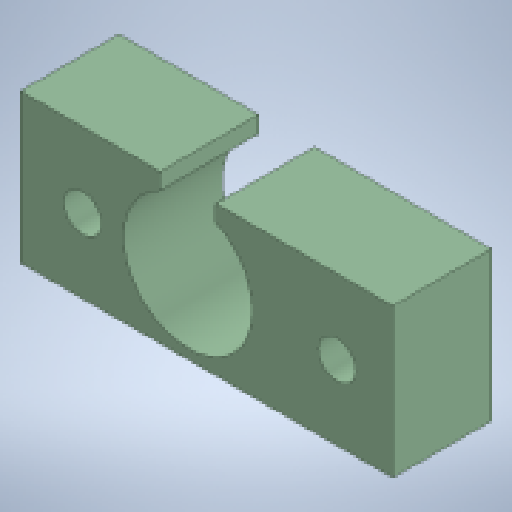
# Autodesk Inventor part: Pod
Saved by Autodesk Inventor 2023.2 (Build 272271000, 271)
## iProperties
Created: 2023-03-29
Part Number: Pod
Material: UHMW, White
Document SubType Name: Modeling
Designer: Nathan Cai
Density: 0.94 g/cm^3
Appearance: Rubber - Green
Author: Nathan Cai
Autodesk Inventor part; units mm, degrees
ref_plane "YZ Plane" through (0, 0, 0) normal (1, 0, 0) x (0, 1, 0)
ref_plane "XZ Plane" through (0, 0, 0) normal (0, 1, 0) x (-1, 0, 0)
ref_plane "XY Plane" through (0, 0, 0) normal (0, 0, 1) x (1, 0, 0)
sketch "Sketch1" plane through (0, 0, 0) normal (0, 0, 1) x (1, 0, 0)
  circle A0 centre (0, 0) radius 11
  line L0 (0, 0) -> (-18, 0) construction
  circle A1 centre (-18, 0) radius 3.175
  circle A2 centre (-18, 0) radius 38.1 construction
  circle A3 centre (25.4, 0) radius 1.7526 construction
  circle A4 centre (25.4, 0) radius 3.175
  line L1 (-23.8125, 12.7) -> (14.2875, 12.7)
  line L2 (14.2875, 12.7) -> (14.2875, -12.7)
  line L3 (14.2875, -12.7) -> (-23.8125, -12.7)
  line L4 (-23.8125, -12.7) -> (-23.8125, 12.7)
  line L5 (-23.8125, 12.7) -> (14.2875, -12.7) construction
  line L6 (14.2875, 12.7) -> (-23.8125, -12.7) construction
  line L7 (-9.525, -9.525) -> (9.525, -9.525) construction
  line L8 (9.525, -9.525) -> (9.525, 9.525) construction
  line L9 (9.525, 9.525) -> (-9.525, 9.525) construction
  line L10 (-9.525, 9.525) -> (-9.525, -9.525) construction
  line L11 (-9.525, -9.525) -> (9.525, 9.525) construction
  line L12 (9.525, -9.525) -> (-9.525, 9.525) construction
  circle A5 centre (-9.525, 9.525) radius 1.7526
  circle A6 centre (9.525, 9.525) radius 1.7526
  circle A7 centre (-9.525, -9.525) radius 1.7526
  circle A8 centre (9.525, -9.525) radius 1.7526
  point P0 (-4.7625, 0)
  dimension "d0" = 22
  dimension "d1" = 18
  dimension "d2" = 6.35
  dimension "d3" = 76.2
  dimension "d4" = 3.5052
  dimension "d5" = 25.4
  dimension "d6" = 6.35
  dimension "d7" = 38.1
  dimension "d8" = 25.4
  dimension "d16" = 4.7625
  dimension "d18" = 19.05
  dimension "d19" = 19.05
  dimension "d20" = 3.5052
  dimension "d23" = 19.05
  dimension "d26" = 19.05
  constraints: 26 end point, 9 centre point, 5 coincident, 4 horizontal, 4 midpoint, 4 parallel, 2 perpendicular, 2 point on line, 1 vertical, 6 other
  measures "d0" diameter of A0
  measures "d1" distance of L0.start L0.end
  measures "d2" diameter of A1
  measures "d3" diameter of A2
  measures "d4" diameter of A3
  measures "d5" distance of point (0, 0) A3.centre
  measures "d6" diameter of A4
  measures "d7" distance of L2.end L3.end
  measures "d8" distance of L1.end L2.end
  measures "d16" distance of point (0, 0) point (-4.763, 0)
  measures "d18" distance of L9.end L8.end
  measures "d19" distance of L8.end L7.end
  measures "d20" diameter of A5
  measures "d23" distance of A5.centre A6.centre
  measures "d26" distance of A5.centre A7.centre
extrude "Extrusion1" add sketch "Sketch1" along normal blind 16.8 contours L1 L2 L3 L4
sketch "Sketch2" plane through (-23.8125, 12.7, 0) normal (0, 1, 0) x (1, 0, 0)
  line L0 (0, -16.8) -> (38.1, -16.8) projected
  line L1 (19.05, -16.8) -> (19.05, 16.8) construction
  line L2 (23.8125, -16.8) -> (23.8125, 0) construction
  line L3 (0, 0) -> (38.1, 0) projected
  line L4 (28.575, -16.8) -> (19.05, -16.8)
  line L5 (19.05, -16.8) -> (19.05, 0)
  line L6 (19.05, 0) -> (28.575, 0)
  line L7 (28.575, 0) -> (28.575, -16.8)
  line L8 (28.575, -16.8) -> (19.05, 0) construction
  line L9 (19.05, -16.8) -> (28.575, 0) construction
  point P0 (23.8125, 0)
  point P1 (23.8125, -8.4)
  dimension "d13" = 9.525
  dimension "d17" = 4.7625
  constraints: 16 end point, 5 midpoint, 2 parallel, 2 vertical, 1 horizontal, 1 perpendicular, 1 point on line, 4 other
  measures "d13" distance of L5.end L6.end
  measures "d17" distance between parallel lines of L1 L2
extrude "Extrusion2" cut sketch "Sketch2" against normal blind 19.05
sketch "Sketch3" plane through (-23.8125, 12.7, 16.8) normal (0, 1, 0) x (1, 0, 0)
  line L0 (0, 0) -> (38.1, 0) projected
  line L1 (38.1, 0) -> (9.525, 0)
  line L2 (9.525, 0) -> (9.525, -22.225)
  line L3 (9.525, -22.225) -> (38.1, -22.225)
  line L4 (38.1, -22.225) -> (38.1, 0)
  line L5 (11.1125, -19.8438) -> (11.1125, 0)
  line L6 (36.5125, 0) -> (36.5125, -19.8437)
  line L7 (36.5125, -19.8437) -> (11.1125, -19.8438)
  point P0 (23.8125, 16.8)
  point P1 (11.1125, 0)
  dimension "d29" = 28.575
  dimension "d30" = 22.225
  dimension "d31" = 1.5875
  dimension "d32" = 2.3813
  constraints: 14 end point, 3 parallel, 2 point on line, 1 horizontal, 1 perpendicular
  measures "d29" distance of L3.end L2.end
  measures "d30" distance of L2.end L1.end
  measures "d31" distance between parallel lines of L2 L5
  measures "d32" distance between parallel lines of L3 L7
extrude "Extrusion3" add sketch "Sketch3" against normal up to surface (25.4 mm away) contours L0 L5 L7 L6 L4 L3 L2
fillet "Fillet1" radius 4.7625 2 edges at (12.7, 0, 36.6437) (-12.7, 0, 36.6438)
fillet "Fillet2" radius 3.175 4 edges at (-12.7, 0, 16.8) (12.7, 0, 16.8) (-14.2875, 0, 39.025) (14.2875, 0, 39.025)
sketch "Sketch4" plane through (-23.8125, 12.7, 16.8) normal (0, 1, 0) x (1, 0, 0)
  line L0 (0, 0) -> (9.525, 0) projected
  line L1 (9.525, 0) -> (22.225, 0)
  line L2 (22.225, 0) -> (22.225, -9.525)
  line L3 (22.225, -9.525) -> (9.525, -9.525)
  line L4 (9.525, -9.525) -> (9.525, 0)
  point P0 (23.8125, 16.8)
  dimension "d37" = 12.7
  dimension "d38" = 9.525
  constraints: 8 end point, 2 parallel, 1 horizontal, 1 perpendicular
  measures "d37" distance of L2.end L3.end
  measures "d38" distance of L1.end L2.end
extrude "Extrusion4" cut sketch "Sketch4" against normal blind 19.05
fillet "Fillet3" radius 4.7625 3 edges at (-11.9062, -6.35, 16.8) (-13.4937, -6.35, 26.325) (-13.4937, 12.7, 26.325)
fillet "Fillet4" radius 3.175 2 edges at (-4.7625, 9.9156, 8.4) (4.7625, 9.9156, 8.4)
sketch "Sketch5" plane through (0, 0, 0) normal (0, 0, -1) x (-1, 0, 0)
  line L0 (-12.7, 12.7) -> (12.7, 12.7)
  line L1 (12.7, 12.7) -> (12.7, -12.7)
  line L2 (12.7, -12.7) -> (-12.7, -12.7)
  line L3 (-12.7, -12.7) -> (-12.7, 12.7)
  line L4 (-12.7, 12.7) -> (12.7, -12.7) construction
  line L5 (12.7, 12.7) -> (-12.7, -12.7) construction
  circle A0 centre (18, 0) radius 3.175 projected
  circle A1 centre (18, 0) radius 5.8125
  line L6 (23.8125, 12.7) -> (23.8125, -12.7) projected
  point P0 (0, 0)
  point P1 (12.7, 2.3865)
  point P2 (12.7, -2.3865)
  dimension "d43" = 25.4
  dimension "d44" = 25.4
  constraints: 12 end point, 2 midpoint, 2 parallel, 1 centre point, 1 coincident, 1 horizontal, 1 perpendicular, 1 tangent
  measures "d43" distance of L1.end L2.end
  measures "d44" distance of L0.end L1.end
equation "\"d23\" = d18"
equation "\"d26\" = d19"
body "Solid1"
